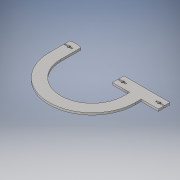
# Autodesk Inventor part: Zoetrope_Hook
Saved by Autodesk Inventor 2016 (Build 200138000, 138)
## iProperties
Created: 2019-03-08
Part Number: Zoetrope_Hook
Material: Generic
Document SubType Name: Modeling
Designer: student
Density: 1 g/cm^3
Appearance: Default
Author: student
Autodesk Inventor part; units mm, degrees
ref_plane "YZ Plane" through (0, 0, 0) normal (1, 0, 0) x (0, 1, 0)
ref_plane "XZ Plane" through (0, 0, 0) normal (0, 1, 0) x (-1, 0, 0)
ref_plane "XY Plane" through (0, 0, 0) normal (0, 0, 1) x (1, 0, 0)
sketch "Sketch1" plane through (0, 0, 0) normal (0, 1, 0) x (-1, 0, 0)
  line L0 (0, 0) -> (114.7109, 0) construction
  line L1 (114.7109, 0) -> (229.0109, 0) construction
  line L2 (63.5, 69.85) -> (63.5, 57.15)
  line L3 (38.1, 69.85) -> (38.1, 57.15)
  line L4 (63.5, 57.15) -> (101.6, 57.15)
  line L5 (38.1, 57.15) -> (0, 57.15)
  line L6 (101.6, 31.75) -> (0, 31.75)
  arc A0 (203.2, 69.85) -> (63.5, 69.85) centre (133.35, 69.85) ccw
  arc A1 (228.6, 69.85) -> (38.1, 69.85) centre (133.35, 69.85) ccw
  line L7 (229.0109, 0) -> (229.0109, 15.875) construction
  line L8 (203.2, 69.85) -> (203.2, 25.0136)
  arc A2 (203.2, 25.0136) -> (228.6, 25.0136) centre (215.9, 62.0354) ccw
  line L9 (228.6, 38.0368) -> (219.3036, 38.0368)
  line L10 (219.3036, 38.0368) -> (219.3036, 39.637)
  line L11 (219.3036, 39.637) -> (216.6366, 39.637)
  line L12 (216.6366, 39.637) -> (216.6366, 38.0368)
  line L13 (216.6366, 38.0368) -> (210.82, 38.0368)
  line L14 (210.82, 38.0368) -> (210.82, 35.3698)
  line L15 (210.82, 35.3698) -> (216.6366, 35.3698)
  line L16 (216.6366, 35.3698) -> (216.6366, 33.7696)
  line L17 (216.6366, 33.7696) -> (219.3036, 33.7696)
  line L18 (219.3036, 33.7696) -> (219.3036, 35.3698)
  line L19 (219.3036, 35.3698) -> (228.6, 35.3698)
  line L20 (101.6, 45.7835) -> (92.3036, 45.7835)
  line L21 (92.3036, 45.7835) -> (92.3036, 47.3837)
  line L22 (92.3036, 47.3837) -> (89.6366, 47.3837)
  line L23 (89.6366, 47.3837) -> (89.6366, 45.7835)
  line L24 (89.6366, 45.7835) -> (83.82, 45.7835)
  line L25 (83.82, 45.7835) -> (83.82, 43.1165)
  line L26 (83.82, 43.1165) -> (89.6366, 43.1165)
  line L27 (89.6366, 43.1165) -> (89.6366, 41.5163)
  line L28 (89.6366, 41.5163) -> (92.3036, 41.5163)
  line L29 (92.3036, 41.5163) -> (92.3036, 43.1165)
  line L30 (92.3036, 43.1165) -> (101.6, 43.1165)
  line L31 (50.8, 31.75) -> (50.8, 58.6536)
  line L32 (0, 45.7835) -> (9.2964, 45.7835)
  line L33 (9.2964, 45.7835) -> (9.2964, 47.3837)
  line L34 (9.2964, 47.3837) -> (11.9634, 47.3837)
  line L35 (11.9634, 47.3837) -> (11.9634, 45.7835)
  line L36 (11.9634, 45.7835) -> (17.78, 45.7835)
  line L37 (17.78, 45.7835) -> (17.78, 43.1165)
  line L38 (17.78, 43.1165) -> (11.9634, 43.1165)
  line L39 (11.9634, 43.1165) -> (11.9634, 41.5163)
  line L40 (11.9634, 41.5163) -> (9.2964, 41.5163)
  line L41 (9.2964, 41.5163) -> (9.2964, 43.1165)
  line L42 (9.2964, 43.1165) -> (0, 43.1165)
  line L43 (101.6, 57.15) -> (101.6, 45.7835)
  line L44 (101.6, 43.1165) -> (101.6, 31.75)
  line L45 (0, 57.15) -> (0, 45.7835)
  line L46 (0, 43.1165) -> (0, 31.75)
  line L47 (228.6, 69.85) -> (228.6, 38.0368)
  line L48 (228.6, 35.3698) -> (228.6, 25.0136)
  dimension "d12" = 12.7
  dimension "d13" = 38.1
  dimension "d15" = 25.4
  dimension "d16" = 25.4
  dimension "d19" = 190.5
  dimension "d20" = 15.875
  dimension "d23" = 1.6002
  dimension "d24" = 2.667
  dimension "d25" = 5.8166
  dimension "d26" = 1.6002
  dimension "d27" = 2.667
  dimension "d28" = 5.8166
  dimension "d29" = 9.2964
  dimension "d33" = 9.2964
  dimension "d34" = 1.6002
  dimension "d35" = 2.667
  dimension "d36" = 5.8166
  dimension "d37" = 1.6002
  dimension "d38" = 95.25
  dimension "d40" = 39.1396
  dimension "d41" = 26.6656
  dimension "d42" = 23.9986
  dimension "d43" = 35.3698
  dimension "d44" = 66.04
  constraints: 98 end point, 12 perpendicular, 12 symmetric about line, 10 vertical, 6 point on circle, 5 horizontal, 4 point on line, 3 centre point, 2 collinear, 2 tangent, 1 midpoint
  measures "d12" distance of L2.start L2.end
  measures "d13" distance of L3.end L5.end
  measures "d15" distance between parallel lines of L6 L4
  measures "d16" distance between parallel lines of L3 L2
  measures "d19" distance of L3.start L47.start
  measures "d20" distance of L1.end L7.end
  measures "d23" distance of L9.end L10.end
  measures "d24" distance of L10.end L11.end
  measures "d25" distance of L12.end L13.end
  measures "d26" distance of L15.end L16.end
  measures "d27" distance of L13.end L14.end
  measures "d28" distance of L14.end L15.end
  measures "d29" distance of L18.end L19.end
  measures "d33" distance of L20.start L20.end
  measures "d34" distance of L20.end L21.end
  measures "d35" distance of L21.end L22.end
  measures "d36" distance of L23.end L24.end
  measures "d37" distance of L26.end L27.end
  measures "d38" radius of A1
  measures "d40" radius of A2
  measures "d41" distance from line of L19 A2.centre
  measures "d42" distance from line of A2.centre L9
  measures "d43" distance between parallel lines of L1 L19
  measures "d44" distance between parallel lines of L25 L37
extrude "Extrusion1" add sketch "Sketch1" along normal blind 4.572
body "Solid1"
